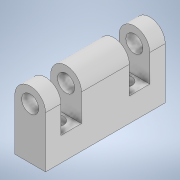
# Autodesk Inventor part: Peça19
Saved by Autodesk Inventor 2021 (Build 250183000, 183)
## iProperties
Created: 2021-07-19
Part Number: Peça19
Material: Genérico
Document SubType Name: Modeling
Designer: Giovanni
Density: 1 g/cm^3
Appearance: Padrão
Author: Giovanni
Autodesk Inventor part; units mm, degrees
ref_plane "YZ Plane" through (0, 0, 0) normal (1, 0, 0) x (0, 1, 0)
ref_plane "XZ Plane" through (0, 0, 0) normal (0, 1, 0) x (-1, 0, 0)
ref_plane "XY Plane" through (0, 0, 0) normal (0, 0, 1) x (1, 0, 0)
sketch "Esboço1" plane through (0, 0, 0) normal (0, 0, 1) x (1, 0, 0)
  arc A0 (9, 0) -> (-9, 0) centre (0, 0) ccw
  line L0 (-9, 0) -> (-9, -30)
  line L1 (-9, -30) -> (9, -30)
  line L2 (9, -30) -> (9, 0)
  dimension "d1" = 9
  dimension "d2" = 30
  constraints: 6 end point, 2 point on circle, 2 vertical, 1 centre point, 1 coincident, 1 perpendicular, 1 tangent
  measures "d1" radius of A0
  measures "d2" distance of L0.start L0.end
extrude "Extrusão1" add sketch "Esboço1" along normal mid plane 70
sketch "Esboço2" plane through (0, 0, 0) normal (1, 0, 0) x (0, 1, 0)
  line L0 (9, -35) -> (9, 35) projected
  line L1 (9, 26) -> (-16, 26)
  line L2 (-16, 26) -> (-16, 14)
  line L3 (-16, 14) -> (9, 14)
  line L4 (9, 14) -> (9, 26)
  line L5 (9, -14) -> (-16, -14)
  line L6 (-16, -14) -> (-16, -26)
  line L7 (-16, -26) -> (9, -26)
  line L8 (9, -26) -> (9, -14)
  line L9 (-30, -35) -> (-30, 35) projected
  point P0 (0, 0)
  point P1 (-16, -20)
  point P2 (-16, 20)
  dimension "d5" = 12
  dimension "d6" = 14
  dimension "d7" = 14
  dimension "d8" = 14
  dimension "d9" = 12
  constraints: 16 end point, 4 parallel, 3 point on line, 2 horizontal, 2 midpoint, 2 perpendicular, 1 vertical alignment
  measures "d5" distance between parallel lines of L3 L1
  measures "d6" distance from line of point (0, 0) L3
  measures "d7" distance between parallel lines of L9 L2
  measures "d8" distance from line of L5 point (0, 0)
  measures "d9" distance between parallel lines of L7 L5
extrude "Extrusão2" cut sketch "Esboço2" along normal mid plane 20
sketch "Esboço3" plane through (0, 0, 35) normal (0, 0, 1) x (1, 0, 0)
  circle A0 centre (0, 0) radius 5
  dimension "d12" = 10
  constraints: 1 centre point, 1 coincident
  measures "d12" diameter of A0
extrude "Extrusão3" cut sketch "Esboço3" against normal through all
sketch "Esboço4" plane through (-9, -16, 26) normal (0, 1, 0) x (1, 0, 0)
  point P0 (9, 26)
  point P1 (9, 6)
  point P2 (9, 46)
  dimension "d15" = 20
  dimension "d16" = 20
  constraints: 2 vertical alignment
  measures "d15" distance of point (9, 26) point (9, 6)
  measures "d16" distance of point (9, 46) point (9, 26)
hole "Furo1" at (0, -16, 20) at (0, -16, -20) direction (0, -1, 0) diameter 5 end through all counterbore diameter 9 counterbore depth 5
